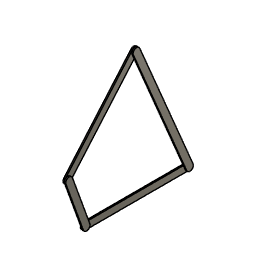
fourbar_mechanism (Autodesk Fusion 360 design; units mm, degrees)
Autodesk Fusion 360 part; units mm, degrees
sketch "Sketch1" plane through (0, 0, 0) normal (1, 0, 0) x (0, 1, 0)
  line L0 (0, -5) -> (75, -5)
  arc A0 (75, -5) -> (75, 5) centre (75, 0) ccw
  line L1 (75, 5) -> (0, 5)
  arc A1 (0, 5) -> (0, -5) centre (0, 0) ccw
  line L2 (0, 0) -> (75, 0) construction
  line L3 (0, -25) -> (150, -25)
  arc A2 (150, -25) -> (150, -15) centre (150, -20) ccw
  line L4 (150, -15) -> (0, -15)
  arc A3 (0, -15) -> (0, -25) centre (0, -20) ccw
  line L5 (0, -20) -> (150, -20) construction
  line L6 (0, -45) -> (150, -45)
  arc A4 (150, -45) -> (150, -35) centre (150, -40) ccw
  line L7 (150, -35) -> (0, -35)
  arc A5 (0, -35) -> (0, -45) centre (0, -40) ccw
  line L8 (0, -40) -> (150, -40) construction
  line L9 (0, -65) -> (200, -65)
  arc A6 (200, -65) -> (200, -55) centre (200, -60) ccw
  line L10 (200, -55) -> (0, -55)
  arc A7 (0, -55) -> (0, -65) centre (0, -60) ccw
  line L11 (0, -60) -> (200, -60) construction
  constraint tangent L0 A0
  constraint tangent A0 L1
  constraint parallel L0 L1
  constraint tangent L1 A1
  constraint tangent L0 A1
  constraint horizontal L2
  constraint coincident A1.centre L2.start
  constraint tangent L3 A2
  constraint tangent A2 L4
  constraint parallel L3 L4
  constraint tangent L4 A3
  constraint tangent L3 A3
  constraint horizontal L5
  constraint tangent L6 A4
  constraint tangent A4 L7
  constraint parallel L6 L7
  constraint tangent L7 A5
  constraint tangent L6 A5
  constraint parallel L4 L8
  constraint tangent L9 A6
  constraint tangent A6 L10
  constraint parallel L9 L10
  constraint tangent L10 A7
  constraint tangent L9 A7
  constraint parallel L0 L11
extrude "Extrude1" add sketch "Sketch1" along normal blind 2 makes body 1 at (0, 50, -21.6667) makes body 2 at (0, 50, -41.6667) makes body 3 at (0, 50, -1.6667) makes body 4 at (0, 133.3333, -61.6667) in component "Component"
copy_body "Body->Comp1" bodies 1 removing the originals makes body 5 in component "Component'"
copy_body "Body->Comp2" bodies 2 removing the originals makes body 6 in component "Component''"
copy_body "Body->Comp3" bodies 3 removing the originals makes body 7 in component "Component'''"
copy_body "Body->Comp4" bodies 4 removing the originals makes body 8 in component "Component''''"
component "Component" placed x (1, 0, 0) y (0, 1, 0) z (0, 0, 1) at (0, 0, 0)
component "Component''" placed x (1, 0, 0) y (0, 0.22487, -0.974389) z (0, 0.974389, 0.22487) at (0, 77.5494, 155.0798) in component "Component"
component "Component'''" placed x (-1, 0, 0) y (0, 0.964059, 0.265689) z (0, 0.265689, -0.964059) at (4, 0, -20) in component "Component"
component "Component''''" placed x (-1, 0, 0) y (0, -0.557131, 0.830425) z (0, 0.830425, 0.557131) at (4, 199.8255, 13.4278) in component "Component"
component "Component'" placed x (1, 0, 0) y (0, 1, 0) z (0, 0, 1) at (0, 0, 0) in component "Component"
